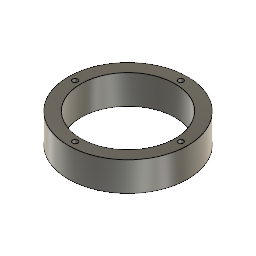
sockel (Autodesk Fusion 360 design; units mm, degrees)
Autodesk Fusion 360 part; units mm, degrees
sketch "Skizze1" plane through (0, 0, 0) normal (0, 0, 1) x (1, 0, 0)
  circle A0 centre (0, 0) radius 45
  circle A1 centre (0, 0) radius 57
  line L0 (-93.8803, 0) -> (101.1197, 0) construction
  line L1 (0, 80) -> (0, -75) construction
  circle A2 centre (50.5, 0) radius 1.45
  circle A3 centre (0, 50.5) radius 1.45
  line L2 (-57, 57) -> (57, 57) construction
  line L3 (57, 57) -> (57, -57) construction
  line L4 (57, -57) -> (-57, -57) construction
  line L5 (-57, -57) -> (-57, 57) construction
  circle A4 centre (50.5, 0) radius 2.45
  circle A5 centre (0, 50.5) radius 2.45
  circle A6 centre (-50.5, 0) radius 2.45
  circle A7 centre (-50.5, 0) radius 1.45
  circle A8 centre (0, -50.5) radius 2.45
  circle A9 centre (0, -50.5) radius 1.45
  dimension "d1" = 90
  dimension "d2" = 114
  dimension "d3" = 2.9
  dimension "d4" = 2.9
  dimension "d5" = 6.5
  dimension "d6" = 6.5
  dimension "d7" = 4.9
  dimension "d8" = 4.9
  measures "d1" diameter of A0
  measures "d2" diameter of A1
  measures "d3" diameter of A2
  measures "d4" diameter of A3
  measures "d7" diameter of A4
  measures "d8" diameter of A5
extrude "Extrusion1" add sketch "Skizze1" along normal blind 28 contours A1
extrude "Extrusion2" add sketch "Skizze1" along normal blind 24.5 contours A4 | A5 | A6 | A8
equation "d4 = d3"
equation "d6 = d5"
equation "d8 = d7"
